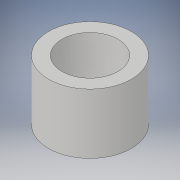
# Autodesk Inventor part: EncoderBush1
Saved by Autodesk Inventor 2018.3 (Build 223284000, 284)
## iProperties
Created: 2018-07-05
Part Number: EncoderBush1
Material: Generisch
Document SubType Name: Modeling
Designer: JochenAlt
Density: 1 g/cm^3
Appearance: Vorgabe
Author: JochenAlt
Autodesk Inventor part; units mm, degrees
ref_plane "YZ Plane" through (0, 0, 0) normal (1, 0, 0) x (0, 1, 0)
ref_plane "XZ Plane" through (0, 0, 0) normal (0, 1, 0) x (-1, 0, 0)
ref_plane "XY Plane" through (0, 0, 0) normal (0, 0, 1) x (1, 0, 0)
sketch "Skizze1" plane through (0, 0, 0) normal (0, 0, 1) x (1, 0, 0)
  circle A0 centre (0, 0) radius 2.1
  circle A1 centre (0, 0) radius 3.1
  dimension "d0" = 4.2
  dimension "d1" = 1
  constraints: 2 centre point, 2 coincident
  measures "d0" diameter of A0
  measures "d1" radial gap between concentric circles of A1 A0
extrude "Extrusion1" add sketch "Skizze1" along normal blind 4.5
